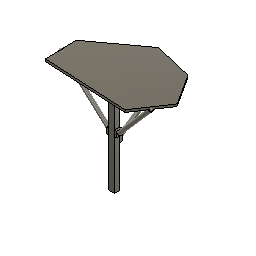
monorail (Autodesk Fusion 360 design; units mm, degrees)
Autodesk Fusion 360 part; units mm, degrees
sketch "Sketch1" plane through (0, 0, 0) normal (0, 1, 0) x (1, 0, 0)
  line L0 (0, 0) -> (-5, 0)
  line L1 (-5, 0) -> (-5, -5)
  line L2 (-5, -5) -> (0, -5)
  line L3 (0, -5) -> (0, 0)
  constraint horizontal L0
  constraint vertical L1
  constraint horizontal L2
  constraint vertical L3
  constraint coincident L0.start L3.end
extrude "Extrude1" add sketch "Sketch1" along normal blind 2.5 makes body 1
extrude "Extrude2" add 1 faces at (-3.3333, 2.5, 1.6667) along direction (0, 1, 0) blind 80 on bodies 1 bodies 1
sketch "Sketch2" plane through (0, 0, 0) normal (0, 0, 1) x (1, 0, 0)
  line L0 (0, 5) -> (2, 5)
  line L1 (2, 5) -> (2, 10)
  line L2 (2, 10) -> (0, 10)
  line L3 (0, 10) -> (0, 5)
  constraint horizontal L0
  constraint vertical L1
  constraint horizontal L2
  constraint vertical L3
extrude "Extrude3" add sketch "Sketch2" along normal blind 5 separate body makes body 2
sphere "SpherePrimitive1" cut diameter 2.5 placed x (0, 0, -1) y (0, 1, 0) z (1, 0, 0) at (2, 7.5, 2.5) bodies 2
cylinder "CylinderPrimitive1" add diameter 3.5 height 45 placed x (1, 0, 0) y (0, 0, -1) z (0, 1, 0) at (15, 0, 0) separate body makes body 3
extrude "Extrude4" add 1 faces at (14.4232, 45, -0.7066) along direction (0, 1, 0) blind 15 on bodies 3 bodies 3
sphere "SpherePrimitive2" add diameter 2.5 placed x (1, 0, 0) y (0, 0, 1) z (0, -1, 0) at (15, 0, 0) bodies 3
sphere "SpherePrimitive3" add diameter 2.5 placed x (-1, 0, 0) y (0, 0, 1) z (0, 1, 0) at (15, 60, 0) bodies 3
copy_body "CopyPasteBodies1" bodies 3 2 makes body 4 makes body 5
move_body "Move1" bodies 4 5 to x (1, 0, 0) y (0, 1, 0) z (0, 0, 1) at (-12.4926, 0, -17.6032)
copy_body "CopyPasteBodies3" bodies 4 makes body 6
move_body "Move2" bodies 6 to x (1, 0, 0) y (0, 1, 0) z (0, 0, 1) at (19.3713, 0, -0.932)
copy_body "CopyPasteBodies4" bodies 5 makes body 7
move_body "Move3" bodies 7 to x (1, 0, 0) y (0, 1, 0) z (0, 0, 1) at (-10.1487, 0, 0)
sketch "Sketch9" plane through (0, 0, 0) normal (0, 1, 0) x (1, 0, 0)
  line L0 (20, 0) -> (0, -25)
  line L1 (0, -25) -> (-22.7284, 8.4291)
  line L2 (-22.7284, 8.4291) -> (20, 0)
  line L3 (11.59, -26.3409) -> (26.0343, -8.2855)
  line L4 (26.0343, -8.2855) -> (16.8582, 12.7941)
  line L5 (16.8582, 12.7941) -> (-32.8132, 15.2024)
  line L6 (-32.8132, 15.2024) -> (-36.4257, -4.8166)
  line L7 (-36.4257, -4.8166) -> (-12.0415, -29.8028)
  line L8 (-12.0415, -29.8028) -> (11.59, -26.3409)
  constraint parallel L0 L3
extrude "Extrude5" add sketch "Sketch9" along normal blind 2 separate body contours L0 L1 L2 | L3 L4 L5 L6 L7 L8 makes body 8
move_body "Move4" bodies 8 to x (1, 0, 0) y (0, 1, 0) z (0, 0, 1) at (0, 105.9344, 0)
scale "Scale1" factor 1.5 about (-36.4257, 107.9344, 4.8166) bodies 8
extrude "Extrude6" cut 1 faces at (2.4083, 107.9344, 8.5043) along direction (0, -1, 0) blind 1 on bodies 8 bodies 8
copy_body "Body->Comp1" bodies 3 removing the originals makes body 9 in component "poleLeft"
copy_body "Body->Comp2" bodies 8 removing the originals makes body 10 in component "FLAT"
copy_body "Body->Comp3" bodies 4 removing the originals makes body 11 in component "poleRight"
copy_body "Body->Comp4" bodies 5 removing the originals makes body 12 in component "gantryRight"
copy_body "Body->Comp5" bodies 2 removing the originals makes body 13 in component "gantryLeft"
copy_body "Body->Comp6" bodies 1 removing the originals makes body 14 in component "mainHole"
copy_body "Body->Comp7" bodies 7 removing the originals makes body 15 in component "gantryBack"
copy_body "Body->Comp8" bodies 6 removing the originals makes body 16 in component "poleBack"
component "poleLeft" placed x (-0.207052, -0.64012, -0.739848) y (-0.164567, -0.722672, 0.671314) z (-0.964389, 0.260752, 0.044288) at (0.6058, 42.7414, 9.0977)
component "FLAT" placed x (0.984217, -0.165213, 0.063421) y (0.164567, 0.722672, -0.671314) z (0.065077, 0.671156, 0.738454) at (-50.1475, -111.1907, 79.6156)
component "poleRight" placed x (0.086144, 0.990664, -0.105664) y (-0.995443, 0.081232, -0.049953) z (-0.040903, 0.109486, 0.993146) at (-7.936, -42.062, 20.2475)
component "gantryRight" placed x (0, 0, -1) y (0, 1, 0) z (1, 0, 0) at (12.6032, 25.6396, -12.4926)
component "gantryLeft" placed x (1, 0, 0) y (0, -1, 0) z (0, 0, -1) at (0, 19.4041, 5)
component "mainHole" placed x (1, 0, 0) y (0, 1, 0) z (0, 0, 1) at (0, 0, 0)
component "gantryBack" placed x (-1, 0, 0) y (0, -1, 0) z (0, 0, 1) at (-27.6413, -34.0053, 17.6032)
component "poleBack" placed x (-0.963962, -0.234326, 0.12597) y (0.244343, -0.9671, 0.070813) z (0.105232, 0.099041, 0.989503) at (25.0407, 18.8666, 18.0845)
named bodies: "mainHole", "gantryLeft", "poleLeft", "poleRight", "gantryRight", "poleBack", "gantryBack", "FLAT"
